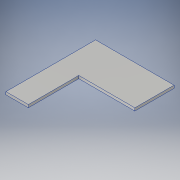
# Autodesk Inventor part: CTU Top
Saved by Autodesk Inventor 2017 (Build 210142000, 142)
## iProperties
Created: 2017-05-04
Part Number: CTU Top
Material: Aluminum 6061
Document SubType Name: Modeling
Designer: qupec
Density: 2.7 g/cm^3
Appearance: Aluminum - Flat
Author: qupec
Autodesk Inventor part; units mm, degrees
ref_plane "YZ Plane" through (0, 0, 0) normal (1, 0, 0) x (0, 1, 0)
ref_plane "XZ Plane" through (0, 0, 0) normal (0, 1, 0) x (-1, 0, 0)
ref_plane "XY Plane" through (0, 0, 0) normal (0, 0, 1) x (1, 0, 0)
sketch "Sketch1" plane through (0, 0, 0) normal (0, 1, 0) x (-1, 0, 0)
  line L0 (88.9, 101.6) -> (38.1, 101.6)
  line L1 (38.1, 101.6) -> (38.1, -12.7)
  line L2 (88.9, -3.6643) -> (88.9, 101.6)
  line L3 (38.1, -12.7) -> (-88.9, -12.7)
  line L4 (-88.9, -12.7) -> (-88.9, -101.6)
  line L5 (-88.9, -101.6) -> (88.9, -101.6)
  line L6 (88.9, -101.6) -> (88.9, -3.6643)
  point P0 (0, 0)
  dimension "d0" = 50.8
  dimension "d1" = 203.2
  dimension "d2" = 177.8
  dimension "d3" = 88.9
  dimension "d4" = 101.6
  dimension "d5" = 88.9
  constraints: 14 end point, 3 parallel, 2 horizontal, 2 perpendicular
  measures "d0" distance between parallel lines of L1 L2
  measures "d1" distance between parallel lines of L0 L5
  measures "d2" distance between parallel lines of L4 L2
  measures "d3" distance between parallel lines of L5 L3
  measures "d4" distance from line of point (0, 0) L0
  measures "d5" distance from line of L4 point (0, 0)
extrude "Extrusion1" add sketch "Sketch1" along normal blind 6.35
equation "\"d4\" = 0.5 * d1"
equation "\"d5\" = 0.5 * d2"
body "Solid1"
